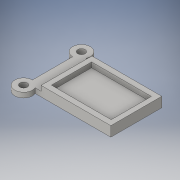
# Autodesk Inventor part: ignition mount
Saved by Autodesk Inventor 2016 (Build 200138000, 138)
## iProperties
Created: 2015-07-08
Part Number: ignition mount
Material: Generic
Document SubType Name: Modeling
Designer: Jacob Kennedy
Density: 1 g/cm^3
Appearance: Default
Author: Jacob Kennedy
Autodesk Inventor part; units mm, degrees
ref_plane "YZ Plane" through (0, 0, 0) normal (1, 0, 0) x (0, 1, 0)
ref_plane "XZ Plane" through (0, 0, 0) normal (0, 1, 0) x (-1, 0, 0)
ref_plane "XY Plane" through (0, 0, 0) normal (0, 0, 1) x (1, 0, 0)
sketch "Sketch1" plane through (0, 0, 0) normal (0, 1, 0) x (-1, 0, 0)
  circle A0 centre (-2.8575, -62.5475) radius 4.699
  circle A1 centre (-2.8575, 11.1125) radius 4.699
  arc A2 (-2.8575, -0.1128) -> (-13.1816, 6.7056) centre (-2.8575, 11.1125) ccw
  arc A3 (-13.1816, -58.1406) -> (-2.8575, -51.3222) centre (-2.8575, -62.5475) ccw
  line L0 (-13.1816, 6.7056) -> (-109.5375, 6.7056)
  line L1 (-109.5375, 6.7056) -> (-109.5375, -58.1406)
  line L2 (-109.5375, -58.1406) -> (-13.1816, -58.1406)
  line L3 (-2.8575, -51.3222) -> (-2.8575, -0.1128)
  line L4 (-2.8575, -0.1128) -> (-2.8575, -51.3222)
  line L5 (-103.1875, -51.3222) -> (-26.9875, -51.3222)
  line L6 (-26.9875, -51.3222) -> (-26.9875, -0.1128)
  line L7 (-26.9875, -0.1128) -> (-103.1875, -0.1128)
  line L8 (-103.1875, -0.1128) -> (-103.1875, -51.3222)
  line L9 (-20.6375, 6.7056) -> (-20.6375, -58.1406)
  point P0 (0, 0)
  dimension "d1" = 9.398
  dimension "d2" = 9.398
  dimension "d4" = 6.35
  constraints: 20 end point, 4 centre point, 4 parallel, 4 point on circle, 3 perpendicular, 2 coincident, 2 horizontal, 2 point on line, 1 vertical
  measures "d1" diameter of A0
  measures "d2" diameter of A1
  measures "d4" distance from line of L1 L5.start
extrude "Extrusion1" add sketch "Sketch1" along normal blind 6.35 contours L3 A3 L2 L9 L0 A2 | L9 L2 L1 L0 | L8 L7 L6 L5
sketch "Sketch2" plane through (0, 6.35, 0) normal (0, 1, 0) x (1, 0, 0)
  line L0 (26.9875, 0.1128) -> (103.1875, 0.1128)
  line L1 (103.1875, 0.1128) -> (103.1875, 51.3222)
  line L2 (103.1875, 51.3222) -> (26.9875, 51.3222)
  line L3 (26.9875, 51.3222) -> (26.9875, 0.1128)
  line L4 (13.1816, -6.7056) -> (109.5375, -6.7056) projected
  line L5 (20.6375, -6.7056) -> (20.6375, 58.7375)
  line L6 (109.5375, 58.1406) -> (13.1816, 58.1406) projected
  line L7 (20.6375, -6.7056) -> (109.5375, -6.7056)
  line L8 (109.5375, -6.7056) -> (109.5375, 58.1406)
  line L9 (109.5375, 58.1406) -> (20.6375, 58.1406)
  line L10 (20.6375, 58.1406) -> (20.6375, -6.7056)
  point P0 (0, 0)
  dimension "d7" = 6.35
  constraints: 18 end point, 4 parallel, 2 horizontal, 2 perpendicular, 1 vertical
  measures "d7" distance between parallel lines of L3 L5
extrude "Extrusion2" add sketch "Sketch2" along normal blind 6.35
body "Solid1"
